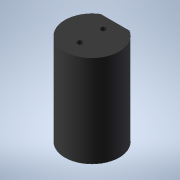
# Autodesk Inventor part: osvesh
Saved by Autodesk Inventor 2020 (Build 240168000, 168)
## iProperties
Created: 2022-10-29
Part Number: osvesh
Material: Типовые
Document SubType Name: Modeling
Designer: akapu
Density: 1 g/cm^3
Appearance: По умолчанию
Author: akapu
Autodesk Inventor part; units mm, degrees
ref_plane "YZ Plane" through (0, 0, 0) normal (1, 0, 0) x (0, 1, 0)
ref_plane "XZ Plane" through (0, 0, 0) normal (0, 1, 0) x (-1, 0, 0)
ref_plane "XY Plane" through (0, 0, 0) normal (0, 0, 1) x (1, 0, 0)
sketch "Эскиз1" plane through (0, 0, 0) normal (0, 1, 0) x (-1, 0, 0)
  circle A0 centre (0, 0) radius 2.95
  circle A1 centre (0, 0) radius 2.5
  line L0 (0, -2.5) -> (1.566, -2.5)
  line L1 (-1.566, -2.5) -> (0, -2.5)
  line L2 (0, 0) -> (0, -1.27)
  line L3 (0, -1.27) -> (0, 1.27)
  circle A2 centre (0, 1.27) radius 0.325
  circle A3 centre (0, -1.27) radius 0.325
  dimension "d1" = 5
  dimension "d0" = 5.9
  dimension "d2" = 1.27
  dimension "d3" = 2.54
  dimension "d4" = 0.65
  dimension "d5" = 0.65
  constraints: 8 end point, 4 coincident, 3 centre point, 3 horizontal, 2 point on circle, 2 point on line, 1 collinear, 1 vertical, 1 vertical alignment, 2 other
  measures "d0" diameter of A0
  measures "d2" distance of L2.start L2.end
  measures "d3" distance of L2.end L3.end
  measures "d4" diameter of A2
  measures "d5" diameter of A3
extrude "Выдавливание1" add sketch "Эскиз1" along normal blind 10 contours A1 | A0 L0 L1 picked at (2.7708, 0.2378)
